Autodesk Fusion 360 part; units mm, degrees
(part 3 of 5)
  line L715 (-40.8866, -85.4677) -> (-40.8866, -98.4677)
  line L716 (118.3697, -66.4177) -> (118.3697, -79.4177)
  arc A698 (151.2072, -3.7177) -> (151.7072, -3.2177) centre (151.2072, -3.2177) ccw
  arc A699 (22.6197, -79.9177) -> (23.1197, -79.4177) centre (22.6197, -79.4177) ccw
  arc A700 (-80.4246, -67.4177) -> (-80.9246, -66.9177) centre (-80.9246, -67.4177) ccw
  line L717 (18.3572, -9.2677) -> (18.3572, -22.2677)
  line L718 (-26.8866, -85.4677) -> (-26.8866, -98.4677)
  arc A701 (155.4629, -62.3677) -> (155.9629, -62.8677) centre (155.9629, -62.3677) ccw
  arc A702 (119.1572, -8.7677) -> (118.6572, -9.2677) centre (119.1572, -9.2677) ccw
  arc A703 (-39.2928, -3.7177) -> (-38.7928, -3.2177) centre (-39.2928, -3.2177) ccw
  line L719 (31.0509, -98.9677) -> (44.0509, -98.9677)
  line L720 (-64.9866, -66.4177) -> (-64.9866, -79.4177)
  line L721 (-87.4246, -67.4177) -> (-87.4246, -81.4177)
  arc A704 (17.8572, -22.7677) -> (18.3572, -22.2677) centre (17.8572, -22.2677) ccw
  arc A705 (-83.7491, -60.3677) -> (-83.2491, -60.8677) centre (-83.2491, -60.3677) ccw
  arc A706 (108.3447, -60.8677) -> (108.8447, -60.3677) centre (108.3447, -60.3677) ccw
  line L722 (176.3072, -65.9177) -> (189.3072, -65.9177)
  line L723 (151.7072, 9.7823) -> (151.7072, -3.2177)
  line L724 (-15.9491, -86.4677) -> (-15.9491, -100.4677)
  arc A707 (-52.2928, -8.7677) -> (-52.7928, -9.2677) centre (-52.2928, -9.2677) ccw
  line L725 (-15.4491, -100.9677) -> (-9.4491, -100.9677)
  line L726 (44.5509, -85.4677) -> (44.5509, -98.4677)
  arc A708 (57.2447, -46.8677) -> (56.7447, -47.3677) centre (57.2447, -47.3677) ccw
  arc A709 (85.3197, -79.4177) -> (85.8197, -79.9177) centre (85.8197, -79.4177) ccw
  line L727 (-48.0303, -66.4177) -> (-48.0303, -79.4177)
  line L728 (80.5572, -9.2677) -> (80.5572, -22.2677)
  arc A710 (-15.4803, -79.9177) -> (-14.9803, -79.4177) centre (-15.4803, -79.4177) ccw
  line L729 (56.4572, -9.2677) -> (56.4572, -22.2677)
  line L730 (138.2072, 10.2823) -> (151.2072, 10.2823)
  arc A711 (-74.5116, -85.4677) -> (-75.0116, -84.9677) centre (-75.0116, -85.4677) ccw
  line L731 (156.7572, 9.7823) -> (156.7572, -3.2177)
  line L732 (47.2197, -66.4177) -> (47.2197, -79.4177)
  arc A712 (9.1197, -79.4177) -> (9.6197, -79.9177) centre (9.6197, -79.4177) ccw
  arc A713 (44.0509, -98.9677) -> (44.5509, -98.4677) centre (44.0509, -98.4677) ccw
  line L733 (-50.6991, -85.4677) -> (-50.6991, -98.4677)
  arc A714 (118.6572, -3.2177) -> (119.1572, -3.7177) centre (119.1572, -3.2177) ccw
  line L734 (100.1072, -8.7677) -> (113.1072, -8.7677)
  line L735 (104.3697, -66.4177) -> (104.3697, -79.4177)
  arc A715 (4.8572, -8.7677) -> (4.3572, -9.2677) centre (4.8572, -9.2677) ccw
  line L736 (186.3389, -48.3677) -> (186.3389, -62.3677)
  arc A716 (99.6072, -3.2177) -> (100.1072, -3.7177) centre (100.1072, -3.2177) ccw
  arc A717 (118.3697, -66.4177) -> (117.8697, -65.9177) centre (117.8697, -66.4177) ccw
  line L737 (28.6697, -65.9177) -> (41.6697, -65.9177)
  arc A718 (60.7197, -79.9177) -> (61.2197, -79.4177) centre (60.7197, -79.4177) ccw
  arc A719 (151.7072, 9.7823) -> (151.2072, 10.2823) centre (151.2072, 9.7823) ccw
  arc A720 (51.1947, -60.8677) -> (51.6947, -60.3677) centre (51.1947, -60.3677) ccw
  arc A721 (117.8697, -79.9177) -> (118.3697, -79.4177) centre (117.8697, -79.4177) ccw
  arc A722 (-40.8866, -98.4677) -> (-40.3866, -98.9677) centre (-40.3866, -98.4677) ccw
  arc A723 (-33.2428, 10.2823) -> (-33.7428, 9.7823) centre (-33.2428, 9.7823) ccw
  arc A724 (66.2697, -79.4177) -> (66.7697, -79.9177) centre (66.7697, -79.4177) ccw
  line L738 (157.2572, 10.2823) -> (170.2572, 10.2823)
  arc A725 (176.3072, -84.9677) -> (175.8072, -85.4677) centre (176.3072, -85.4677) ccw
  arc A726 (-64.1991, -84.9677) -> (-64.6991, -85.4677) centre (-64.1991, -85.4677) ccw
  arc A727 (-64.9866, -66.4177) -> (-65.4866, -65.9177) centre (-65.4866, -66.4177) ccw
  line L739 (-80.4246, -67.4177) -> (-80.4246, -81.4177)
  arc A728 (3.5697, -79.9177) -> (4.0697, -79.4177) centre (3.5697, -79.4177) ccw
  arc A729 (-58.3428, -3.7177) -> (-57.8428, -3.2177) centre (-58.3428, -3.2177) ccw
  arc A730 (-28.4803, -65.9177) -> (-28.9803, -66.4177) centre (-28.4803, -66.4177) ccw
  line L740 (100.1072, -3.7177) -> (113.1072, -3.7177)
  arc A731 (-5.9553, -60.8677) -> (-5.4553, -60.3677) centre (-5.9553, -60.3677) ccw
  arc A732 (-88.0116, -84.9677) -> (-88.5116, -85.4677) centre (-88.0116, -85.4677) ccw
  line L741 (37.4072, -9.2677) -> (37.4072, -22.2677)
  arc A733 (51.6947, -47.3677) -> (51.1947, -46.8677) centre (51.1947, -47.3677) ccw
  arc A734 (19.1447, -46.8677) -> (18.6447, -47.3677) centre (19.1447, -47.3677) ccw
  arc A735 (51.9822, -41.3177) -> (52.4822, -41.8177) centre (52.4822, -41.3177) ccw
  line L742 (99.3197, -66.4177) -> (99.3197, -79.4177)
  line L743 (-19.7428, -9.2677) -> (-19.7428, -22.2677)
  line L744 (47.7197, -65.9177) -> (60.7197, -65.9177)
  line L745 (52.4822, -41.8177) -> (65.4822, -41.8177)
  line L746 (52.4822, -27.8177) -> (65.4822, -27.8177)
  arc A736 (170.2572, -3.7177) -> (170.7572, -3.2177) centre (170.2572, -3.2177) ccw
  line L747 (189.8072, 9.7823) -> (189.8072, -3.2177)
  arc A737 (180.2822, -9.2677) -> (179.7822, -8.7677) centre (179.7822, -9.2677) ccw
  line L748 (208.8572, 9.7823) -> (208.8572, -3.2177)
  arc A738 (208.8572, 9.7823) -> (208.3572, 10.2823) centre (208.3572, 9.7823) ccw
  arc A739 (195.3572, 10.2823) -> (194.8572, 9.7823) centre (195.3572, 9.7823) ccw
  arc A740 (182.2202, -9.7677) -> (181.7202, -10.2677) centre (182.2202, -10.2677) ccw
  arc A741 (208.3572, -3.7177) -> (208.8572, -3.2177) centre (208.3572, -3.2177) ccw
  line L749 (195.3572, 10.2823) -> (208.3572, 10.2823)
  line L750 (195.3572, -3.7177) -> (208.3572, -3.7177)
  line L751 (176.3072, -3.7177) -> (189.3072, -3.7177)
  line L752 (176.3072, 10.2823) -> (189.3072, 10.2823)
  arc A742 (175.8072, -3.2177) -> (176.3072, -3.7177) centre (176.3072, -3.2177) ccw
  arc A743 (195.3572, -8.7677) -> (194.8572, -9.2677) centre (195.3572, -9.2677) ccw
  arc A744 (176.3072, 10.2823) -> (175.8072, 9.7823) centre (176.3072, 9.7823) ccw
  line L753 (195.3572, -8.7677) -> (208.3572, -8.7677)
  arc A745 (170.7572, 9.7823) -> (170.2572, 10.2823) centre (170.2572, 9.7823) ccw
  arc A746 (177.9009, -47.3677) -> (177.4009, -46.8677) centre (177.4009, -47.3677) ccw
  arc A747 (208.8572, -28.3177) -> (208.3572, -27.8177) centre (208.3572, -28.3177) ccw
  arc A748 (171.5447, -27.8177) -> (171.0447, -28.3177) centre (171.5447, -28.3177) ccw
  line L754 (146.9447, -47.3677) -> (146.9447, -60.3677)
  arc A749 (188.2202, -24.7677) -> (188.7202, -24.2677) centre (188.2202, -24.2677) ccw
  line L755 (171.0447, -28.3177) -> (171.0447, -41.3177)
  line L756 (-5.4553, -47.3677) -> (-5.4553, -60.3677)
  arc A750 (195.3572, -27.8177) -> (194.8572, -28.3177) centre (195.3572, -28.3177) ccw
  arc A751 (162.4629, -48.3677) -> (161.9629, -47.8677) centre (161.9629, -48.3677) ccw
  line L757 (208.8572, -9.2677) -> (208.8572, -22.2677)
  line L758 (132.9447, -47.3677) -> (132.9447, -60.3677)
  arc A752 (195.3572, -46.8677) -> (194.8572, -47.3677) centre (195.3572, -47.3677) ccw
  line L759 (180.2822, -9.2677) -> (180.2822, -22.2677)
  arc A753 (186.3389, -48.3677) -> (185.8389, -47.8677) centre (185.8389, -48.3677) ccw
  line L760 (181.7202, -10.2677) -> (181.7202, -24.2677)
  line L761 (-24.5053, -47.3677) -> (-24.5053, -60.3677)
  line L762 (-113.7226, -118.8427) -> (-113.7226, 57.4273)
  line L763 (42.9572, 10.2823) -> (55.9572, 10.2823)
  line L764 (188.7202, -10.2677) -> (188.7202, -24.2677)
  arc A754 (37.4072, -9.2677) -> (36.9072, -8.7677) centre (36.9072, -9.2677) ccw
  line L765 (-43.5553, -47.3677) -> (-43.5553, -60.3677)
  line L766 (194.8572, -9.2677) -> (194.8572, -22.2677)
  line L767 (75.7947, -47.3677) -> (75.7947, -60.3677)
  line L768 (-57.5553, -47.3677) -> (-57.5553, -60.3677)
  line L769 (194.8572, -47.3677) -> (194.8572, -60.3677)
  line L770 (42.9572, -3.7177) -> (55.9572, -3.7177)
  line L771 (177.9009, -47.3677) -> (177.9009, -60.3677)
  arc A755 (55.9572, -3.7177) -> (56.4572, -3.2177) centre (55.9572, -3.2177) ccw
  arc A756 (56.4572, 9.7823) -> (55.9572, 10.2823) centre (55.9572, 9.7823) ccw
  arc A757 (17.8572, -3.7177) -> (18.3572, -3.2177) centre (17.8572, -3.2177) ccw
  line L772 (194.8572, 9.7823) -> (194.8572, -3.2177)
  arc A758 (194.8572, -3.2177) -> (195.3572, -3.7177) centre (195.3572, -3.2177) ccw
  line L773 (175.8072, 9.7823) -> (175.8072, -3.2177)
  arc A759 (188.7202, -10.2677) -> (188.2202, -9.7677) centre (188.2202, -10.2677) ccw
  arc A760 (208.8572, -47.3677) -> (208.3572, -46.8677) centre (208.3572, -47.3677) ccw
  line L774 (171.5447, -27.8177) -> (184.5447, -27.8177)
  arc A761 (179.7822, -22.7677) -> (180.2822, -22.2677) centre (179.7822, -22.2677) ccw
  line L775 (163.9009, -47.3677) -> (163.9009, -60.3677)
  line L776 (195.3572, -46.8677) -> (208.3572, -46.8677)
  line L777 (94.8447, -47.3677) -> (94.8447, -60.3677)
  line L778 (182.2202, -24.7677) -> (188.2202, -24.7677)
  line L779 (179.8389, -47.8677) -> (185.8389, -47.8677)
  line L780 (208.8572, -28.3177) -> (208.8572, -41.3177)
  arc A762 (184.5447, -41.8177) -> (185.0447, -41.3177) centre (184.5447, -41.3177) ccw
  arc A763 (185.0447, -28.3177) -> (184.5447, -27.8177) centre (184.5447, -28.3177) ccw
  arc A764 (189.3072, -3.7177) -> (189.8072, -3.2177) centre (189.3072, -3.2177) ccw
  arc A765 (189.8072, 9.7823) -> (189.3072, 10.2823) centre (189.3072, 9.7823) ccw
  line L781 (182.2202, -9.7677) -> (188.2202, -9.7677)
  line L782 (47.7197, -79.9177) -> (60.7197, -79.9177)
  line L783 (57.2447, -46.8677) -> (70.2447, -46.8677)
  line L784 (-113.7226, 57.4273) -> (228.9474, 57.4273)
  line L785 (18.6447, -47.3677) -> (18.6447, -60.3677)
  line L786 (89.7947, -47.3677) -> (89.7947, -60.3677)
  arc A766 (36.9072, -3.7177) -> (37.4072, -3.2177) centre (36.9072, -3.2177) ccw
  arc A767 (42.9572, -8.7677) -> (42.4572, -9.2677) centre (42.9572, -9.2677) ccw
  line L787 (56.7447, -47.3677) -> (56.7447, -60.3677)
  line L788 (51.6947, -47.3677) -> (51.6947, -60.3677)
  line L789 (-0.4053, -47.3677) -> (-0.4053, -60.3677)
  line L790 (208.8572, -47.3677) -> (208.8572, -60.3677)
  arc A768 (37.4072, 9.7823) -> (36.9072, 10.2823) centre (36.9072, 9.7823) ccw
  line L791 (13.5947, -47.3677) -> (13.5947, -60.3677)
  line L792 (-83.7491, -47.3677) -> (-83.7491, -60.3677)
  line L793 (-38.5053, -47.3677) -> (-38.5053, -60.3677)
  line L794 (127.8947, -47.3677) -> (127.8947, -60.3677)
  line L795 (37.6947, -47.3677) -> (37.6947, -60.3677)
  arc A769 (23.9072, -8.7677) -> (23.4072, -9.2677) centre (23.9072, -9.2677) ccw
  arc A770 (179.8389, -47.8677) -> (179.3389, -48.3677) centre (179.8389, -48.3677) ccw
  line L796 (70.7447, -47.3677) -> (70.7447, -60.3677)
  line L797 (-19.4553, -47.3677) -> (-19.4553, -60.3677)
  arc A771 (56.4572, -9.2677) -> (55.9572, -8.7677) centre (55.9572, -9.2677) ccw
  line L798 (113.8947, -47.3677) -> (113.8947, -60.3677)
  arc A772 (23.9072, 10.2823) -> (23.4072, 9.7823) centre (23.9072, 9.7823) ccw
  line L799 (108.8447, -47.3677) -> (108.8447, -60.3677)
  line L800 (-69.7491, -47.3677) -> (-69.7491, -60.3677)
  line L801 (32.6447, -47.3677) -> (32.6447, -60.3677)
  line L802 (-18.9553, -60.8677) -> (-5.9553, -60.8677)
  line L803 (-23.7178, -27.8177) -> (-10.7178, -27.8177)
  line L804 (228.9474, 57.4273) -> (228.9474, -118.8427)
  arc A773 (18.3572, -9.2677) -> (17.8572, -8.7677) centre (17.8572, -9.2677) ccw
  line L805 (-28.4803, -65.9177) -> (-15.4803, -65.9177)
  line L806 (-33.2428, 10.2823) -> (-20.2428, 10.2823)
  arc A774 (42.4572, -3.2177) -> (42.9572, -3.7177) centre (42.9572, -3.2177) ccw
  line L807 (23.9072, -8.7677) -> (36.9072, -8.7677)
  line L808 (-33.2428, -8.7677) -> (-20.2428, -8.7677)
  line L809 (42.4572, 9.7823) -> (42.4572, -3.2177)
  line L810 (-23.7178, -41.8177) -> (-10.7178, -41.8177)
  line L811 (18.3572, 9.7823) -> (18.3572, -3.2177)
  line L812 (119.1572, -8.7677) -> (132.1572, -8.7677)
  arc A775 (155.9629, -47.8677) -> (155.4629, -48.3677) centre (155.9629, -48.3677) ccw
  line L813 (-28.4803, -79.9177) -> (-15.4803, -79.9177)
  line L814 (123.9197, -79.9177) -> (136.9197, -79.9177)
  line L815 (-57.0553, -60.8677) -> (-44.0553, -60.8677)
  line L816 (128.6822, -27.8177) -> (141.6822, -27.8177)
  line L817 (-64.1991, -98.9677) -> (-51.1991, -98.9677)
  line L818 (-64.1991, -84.9677) -> (-51.1991, -84.9677)
  line L819 (128.6822, -41.8177) -> (141.6822, -41.8177)
  line L820 (42.9572, -8.7677) -> (55.9572, -8.7677)
  line L821 (9.6197, -79.9177) -> (22.6197, -79.9177)
  line L822 (19.1447, -60.8677) -> (32.1447, -60.8677)
  line L823 (-33.2428, -22.7677) -> (-20.2428, -22.7677)
  line L824 (133.4447, -60.8677) -> (146.4447, -60.8677)
  arc A776 (157.2572, 10.2823) -> (156.7572, 9.7823) centre (157.2572, 9.7823) ccw
  line L825 (123.9197, -65.9177) -> (136.9197, -65.9177)
  line L826 (9.6197, -65.9177) -> (22.6197, -65.9177)
  line L827 (119.1572, -22.7677) -> (132.1572, -22.7677)
  line L828 (119.1572, -3.7177) -> (132.1572, -3.7177)
  line L829 (28.6697, -79.9177) -> (41.6697, -79.9177)
  line L830 (119.1572, 10.2823) -> (132.1572, 10.2823)
  line L831 (85.8197, -65.9177) -> (98.8197, -65.9177)
  line L832 (37.4072, 9.7823) -> (37.4072, -3.2177)
  line L833 (138.2072, -8.7677) -> (151.2072, -8.7677)
  line L834 (4.8572, -8.7677) -> (17.8572, -8.7677)
  line L835 (-9.4303, -79.9177) -> (3.5697, -79.9177)
  line L836 (-9.9303, -66.4177) -> (-9.9303, -79.4177)
  arc A777 (-44.0553, -60.8677) -> (-43.5553, -60.3677) centre (-44.0553, -60.3677) ccw
  line L837 (-78.9866, -66.4177) -> (-78.9866, -79.4177)
  line L838 (-15.4491, -85.9677) -> (-9.4491, -85.9677)
  line L839 (-86.9246, -66.9177) -> (-80.9246, -66.9177)
  arc A778 (132.6572, -9.2677) -> (132.1572, -8.7677) centre (132.1572, -9.2677) ccw
  arc A779 (85.8197, -65.9177) -> (85.3197, -66.4177) centre (85.8197, -66.4177) ccw
  arc A780 (-64.6991, -98.4677) -> (-64.1991, -98.9677) centre (-64.1991, -98.4677) ccw
  arc A781 (28.1697, -79.4177) -> (28.6697, -79.9177) centre (28.6697, -79.4177) ccw
  arc A782 (-56.5486, -67.4177) -> (-57.0486, -66.9177) centre (-57.0486, -67.4177) ccw
  arc A783 (56.7447, -60.3677) -> (57.2447, -60.8677) centre (57.2447, -60.3677) ccw
  line L840 (-71.3428, 10.2823) -> (-58.3428, 10.2823)
  line L841 (-9.4303, -65.9177) -> (3.5697, -65.9177)
  arc A784 (156.7572, -3.2177) -> (157.2572, -3.7177) centre (157.2572, -3.2177) ccw
  line L842 (4.8572, 10.2823) -> (17.8572, 10.2823)
  line L843 (31.0509, -84.9677) -> (44.0509, -84.9677)
  line L844 (-88.0116, -98.9677) -> (-75.0116, -98.9677)
  arc A785 (32.1447, -60.8677) -> (32.6447, -60.3677) centre (32.1447, -60.3677) ccw
  arc A786 (44.5509, -85.4677) -> (44.0509, -84.9677) centre (44.0509, -85.4677) ccw
  line L845 (56.4572, 9.7823) -> (56.4572, -3.2177)
  arc A787 (189.3072, -79.9177) -> (189.8072, -79.4177) centre (189.3072, -79.4177) ccw
  arc A788 (-28.9803, -79.4177) -> (-28.4803, -79.9177) centre (-28.4803, -79.4177) ccw
  line L846 (28.1697, -66.4177) -> (28.1697, -79.4177)
  arc A789 (175.8072, -79.4177) -> (176.3072, -79.9177) centre (176.3072, -79.4177) ccw
  arc A790 (66.7697, -65.9177) -> (66.2697, -66.4177) centre (66.7697, -66.4177) ccw
  arc A791 (99.3197, -66.4177) -> (98.8197, -65.9177) centre (98.8197, -66.4177) ccw
  arc A792 (47.2197, -79.4177) -> (47.7197, -79.9177) centre (47.7197, -79.4177) ccw
  line L847 (23.4072, -9.2677) -> (23.4072, -22.2677)
  line L848 (-47.5303, -65.9177) -> (-34.5303, -65.9177)
  arc A793 (37.6947, -60.3677) -> (38.1947, -60.8677) centre (38.1947, -60.3677) ccw
  arc A794 (23.1197, -66.4177) -> (22.6197, -65.9177) centre (22.6197, -66.4177) ccw
  arc A795 (137.7072, -3.2177) -> (138.2072, -3.7177) centre (138.2072, -3.2177) ccw
  arc A796 (208.3572, -79.9177) -> (208.8572, -79.4177) centre (208.3572, -79.4177) ccw
  arc A797 (-63.0486, -66.9177) -> (-63.5486, -67.4177) centre (-63.0486, -67.4177) ccw
  line L849 (99.6072, -9.2677) -> (99.6072, -22.2677)
  line L850 (30.5509, -85.4677) -> (30.5509, -98.4677)
  arc A798 (194.8572, -79.4177) -> (195.3572, -79.9177) centre (195.3572, -79.4177) ccw
  arc A799 (31.0509, -84.9677) -> (30.5509, -85.4677) centre (31.0509, -85.4677) ccw
  arc A800 (-86.9246, -66.9177) -> (-87.4246, -67.4177) centre (-86.9246, -67.4177) ccw
  arc A801 (-14.9803, -66.4177) -> (-15.4803, -65.9177) centre (-15.4803, -66.4177) ccw
  line L851 (-28.9803, -66.4177) -> (-28.9803, -79.4177)
  line L852 (138.2072, -3.7177) -> (151.2072, -3.7177)
  line L853 (0.0947, -60.8677) -> (13.0947, -60.8677)
  arc A802 (-75.0116, -98.9677) -> (-74.5116, -98.4677) centre (-75.0116, -98.4677) ccw
  arc A803 (42.1697, -66.4177) -> (41.6697, -65.9177) centre (41.6697, -66.4177) ccw
  arc A804 (158.3442, -9.7677) -> (157.8442, -10.2677) centre (158.3442, -10.2677) ccw
  arc A805 (132.9447, -60.3677) -> (133.4447, -60.8677) centre (133.4447, -60.3677) ccw
  line L854 (-63.0486, -81.9177) -> (-57.0486, -81.9177)
  line L855 (-14.6928, -9.2677) -> (-14.6928, -22.2677)
  line L856 (-88.5116, -85.4677) -> (-88.5116, -98.4677)
  line L857 (164.4009, -46.8677) -> (177.4009, -46.8677)
  line L858 (-86.9246, -81.9177) -> (-80.9246, -81.9177)
  line L859 (23.1197, -66.4177) -> (23.1197, -79.4177)
  arc A806 (-0.4053, -60.3677) -> (0.0947, -60.8677) centre (0.0947, -60.3677) ccw
  arc A807 (98.8197, -79.9177) -> (99.3197, -79.4177) centre (98.8197, -79.4177) ccw
  line L860 (61.5072, -9.2677) -> (61.5072, -22.2677)
  line L861 (-64.6991, -85.4677) -> (-64.6991, -98.4677)
  arc A808 (-65.4866, -79.9177) -> (-64.9866, -79.4177) centre (-65.4866, -79.4177) ccw
  arc A809 (132.6572, 9.7823) -> (132.1572, 10.2823) centre (132.1572, 9.7823) ccw
  arc A810 (-27.3866, -98.9677) -> (-26.8866, -98.4677) centre (-27.3866, -98.4677) ccw
  arc A811 (47.7197, -65.9177) -> (47.2197, -66.4177) centre (47.7197, -66.4177) ccw
  arc A812 (138.2072, -8.7677) -> (137.7072, -9.2677) centre (138.2072, -9.2677) ccw
  arc A813 (18.3572, 9.7823) -> (17.8572, 10.2823) centre (17.8572, 9.7823) ccw
  arc A814 (28.6697, -65.9177) -> (28.1697, -66.4177) centre (28.6697, -66.4177) ccw
  line L862 (-71.3428, -8.7677) -> (-58.3428, -8.7677)
  line L863 (-71.3428, -3.7177) -> (-58.3428, -3.7177)
  arc A815 (42.9572, 10.2823) -> (42.4572, 9.7823) centre (42.9572, 9.7823) ccw
  line L864 (164.4009, -60.8677) -> (177.4009, -60.8677)
  line L865 (81.0572, 10.2823) -> (94.0572, 10.2823)
  line L866 (157.2572, -3.7177) -> (170.2572, -3.7177)
  line L867 (81.0572, -8.7677) -> (94.0572, -8.7677)
  line L868 (38.1947, -60.8677) -> (51.1947, -60.8677)
  arc A816 (132.1572, -3.7177) -> (132.6572, -3.2177) centre (132.1572, -3.2177) ccw
  arc A817 (-87.4246, -81.4177) -> (-86.9246, -81.9177) centre (-86.9246, -81.4177) ccw
  arc A818 (164.8442, -10.2677) -> (164.3442, -9.7677) centre (164.3442, -10.2677) ccw
  arc A819 (-8.9491, -86.4677) -> (-9.4491, -85.9677) centre (-9.4491, -86.4677) ccw
  arc A820 (13.0947, -60.8677) -> (13.5947, -60.3677) centre (13.0947, -60.3677) ccw
  line L869 (95.3447, -60.8677) -> (108.3447, -60.8677)
  line L870 (-38.0053, -60.8677) -> (-25.0053, -60.8677)
  arc A821 (-80.9246, -81.9177) -> (-80.4246, -81.4177) centre (-80.9246, -81.4177) ccw
  line L871 (90.5822, -27.8177) -> (103.5822, -27.8177)
  arc A822 (-57.0486, -81.9177) -> (-56.5486, -81.4177) centre (-57.0486, -81.4177) ccw
  line L872 (166.7822, -8.7677) -> (179.7822, -8.7677)
  line L873 (-33.2428, -3.7177) -> (-20.2428, -3.7177)
  line L874 (132.6572, 9.7823) -> (132.6572, -3.2177)
  line L875 (23.4072, 9.7823) -> (23.4072, -3.2177)
  line L876 (-61.8178, -27.8177) -> (-48.8178, -27.8177)
  line L877 (81.0572, -3.7177) -> (94.0572, -3.7177)
  line L878 (23.9072, -3.7177) -> (36.9072, -3.7177)
  arc A823 (41.6697, -79.9177) -> (42.1697, -79.4177) centre (41.6697, -79.4177) ccw
  line L879 (90.5822, -41.8177) -> (103.5822, -41.8177)
  arc A824 (-63.5486, -81.4177) -> (-63.0486, -81.9177) centre (-63.0486, -81.4177) ccw
  line L880 (-40.3866, -98.9677) -> (-27.3866, -98.9677)
  arc A825 (-25.0053, -60.8677) -> (-24.5053, -60.3677) centre (-25.0053, -60.3677) ccw
  line L881 (137.7072, 9.7823) -> (137.7072, -3.2177)
  line L882 (4.8572, -3.7177) -> (17.8572, -3.7177)
  line L883 (14.3822, -41.8177) -> (27.3822, -41.8177)
  line L884 (4.8572, -22.7677) -> (17.8572, -22.7677)
  arc A826 (23.4072, -3.2177) -> (23.9072, -3.7177) centre (23.9072, -3.2177) ccw
  line L885 (-47.5303, -79.9177) -> (-34.5303, -79.9177)
  line L886 (85.8197, -79.9177) -> (98.8197, -79.9177)
  line L887 (81.0572, -22.7677) -> (94.0572, -22.7677)
  line L888 (-56.5486, -67.4177) -> (-56.5486, -81.4177)
  arc A827 (-9.9303, -79.4177) -> (-9.4303, -79.9177) centre (-9.4303, -79.4177) ccw
  line L889 (23.9072, 10.2823) -> (36.9072, 10.2823)
  line L890 (-34.0303, -66.4177) -> (-34.0303, -79.4177)
  line L891 (14.3822, -27.8177) -> (27.3822, -27.8177)
  arc A828 (194.8572, -41.3177) -> (195.3572, -41.8177) centre (195.3572, -41.3177) ccw
  arc A829 (194.8572, -22.2677) -> (195.3572, -22.7677) centre (195.3572, -22.2677) ccw
  line L892 (194.8572, -28.3177) -> (194.8572, -41.3177)
  line L893 (195.3572, -22.7677) -> (208.3572, -22.7677)
  arc A830 (208.3572, -41.8177) -> (208.8572, -41.3177) centre (208.3572, -41.3177) ccw
  line L894 (185.0447, -28.3177) -> (185.0447, -41.3177)
  line L895 (195.3572, -41.8177) -> (208.3572, -41.8177)
  arc A831 (181.7202, -24.2677) -> (182.2202, -24.7677) centre (182.2202, -24.2677) ccw
  arc A832 (208.3572, -22.7677) -> (208.8572, -22.2677) centre (208.3572, -22.2677) ccw
  line L896 (171.5447, -41.8177) -> (184.5447, -41.8177)
  arc A833 (171.0447, -41.3177) -> (171.5447, -41.8177) centre (171.5447, -41.3177) ccw
  line L897 (195.3572, -27.8177) -> (208.3572, -27.8177)
  line L898 (57.2447, -60.8677) -> (70.2447, -60.8677)
  line L899 (228.9474, -118.8427) -> (-113.7226, -118.8427)
  line L900 (123.1322, -28.3177) -> (123.1322, -41.3177)
  arc A834 (114.3947, -46.8677) -> (113.8947, -47.3677) centre (114.3947, -47.3677) ccw
  line L901 (156.7572, -85.4677) -> (156.7572, -98.4677)
  line L902 (151.7072, -85.4677) -> (151.7072, -98.4677)
  arc A835 (-71.8428, -22.2677) -> (-71.3428, -22.7677) centre (-71.3428, -22.2677) ccw
  line L903 (-57.0553, -46.8677) -> (-44.0553, -46.8677)
  arc A836 (-69.7491, -47.3677) -> (-70.2491, -46.8677) centre (-70.2491, -47.3677) ccw
  arc A837 (-90.8928, -22.2677) -> (-90.3928, -22.7677) centre (-90.3928, -22.2677) ccw
  arc A838 (170.2572, -98.9677) -> (170.7572, -98.4677) centre (170.2572, -98.4677) ccw
  arc A839 (-86.1303, -41.3177) -> (-85.6303, -41.8177) centre (-85.6303, -41.3177) ccw
  arc A840 (149.6134, -79.4177) -> (150.1134, -79.9177) centre (150.1134, -79.4177) ccw
  arc A841 (-85.6303, -27.8177) -> (-86.1303, -28.3177) centre (-85.6303, -28.3177) ccw
  line L904 (8.8322, -28.3177) -> (8.8322, -41.3177)
  arc A842 (-77.3928, -22.7677) -> (-76.8928, -22.2677) centre (-77.3928, -22.2677) ccw
  line L905 (95.3447, -46.8677) -> (108.3447, -46.8677)
  line L906 (-29.2678, -28.3177) -> (-29.2678, -41.3177)
  arc A843 (-38.0053, -46.8677) -> (-38.5053, -47.3677) centre (-38.0053, -47.3677) ccw
  line L907 (-85.6303, -27.8177) -> (-72.6303, -27.8177)
  arc A844 (163.1134, -79.9177) -> (163.6134, -79.4177) centre (163.1134, -79.4177) ccw
  arc A845 (-33.7428, -22.2677) -> (-33.2428, -22.7677) centre (-33.2428, -22.2677) ccw
  line L908 (114.3947, -46.8677) -> (127.3947, -46.8677)
  arc A846 (14.3822, -27.8177) -> (13.8822, -28.3177) centre (14.3822, -28.3177) ccw
  arc A847 (-58.3428, -22.7677) -> (-57.8428, -22.2677) centre (-58.3428, -22.2677) ccw
  arc A848 (161.9629, -62.8677) -> (162.4629, -62.3677) centre (161.9629, -62.3677) ccw
  line L909 (-85.6303, -41.8177) -> (-72.6303, -41.8177)
  arc A849 (-42.7678, -27.8177) -> (-43.2678, -28.3177) centre (-42.7678, -28.3177) ccw
  arc A850 (163.9009, -60.3677) -> (164.4009, -60.8677) centre (164.4009, -60.3677) ccw
  line L910 (-18.9553, -46.8677) -> (-5.9553, -46.8677)
  arc A851 (-29.2678, -28.3177) -> (-29.7678, -27.8177) centre (-29.7678, -28.3177) ccw
  arc A852 (-4.6678, -27.8177) -> (-5.1678, -28.3177) centre (-4.6678, -28.3177) ccw
  line L911 (137.4197, -66.4177) -> (137.4197, -79.4177)
  line L912 (163.6134, -66.4177) -> (163.6134, -79.4177)
  arc A853 (-83.2491, -46.8677) -> (-83.7491, -47.3677) centre (-83.2491, -47.3677) ccw
  arc A854 (146.4447, -60.8677) -> (146.9447, -60.3677) centre (146.4447, -60.3677) ccw
  line L913 (170.7572, -85.4677) -> (170.7572, -98.4677)
  line L914 (157.2572, -84.9677) -> (170.2572, -84.9677)
  arc A855 (-39.2928, -22.7677) -> (-38.7928, -22.2677) centre (-39.2928, -22.2677) ccw
  arc A856 (-24.2178, -41.3177) -> (-23.7178, -41.8177) centre (-23.7178, -41.3177) ccw
  arc A857 (-29.7678, -41.8177) -> (-29.2678, -41.3177) centre (-29.7678, -41.3177) ccw
  arc A858 (-48.8178, -41.8177) -> (-48.3178, -41.3177) centre (-48.8178, -41.3177) ccw
  arc A859 (151.2072, -98.9677) -> (151.7072, -98.4677) centre (151.2072, -98.4677) ccw
  arc A860 (-43.5553, -47.3677) -> (-44.0553, -46.8677) centre (-44.0553, -47.3677) ccw
  arc A861 (208.8572, -9.2677) -> (208.3572, -8.7677) centre (208.3572, -9.2677) ccw
  line L915 (170.7572, 9.7823) -> (170.7572, -3.2177)
  arc A862 (-72.1303, -28.3177) -> (-72.6303, -27.8177) centre (-72.6303, -28.3177) ccw
  arc A863 (0.0947, -46.8677) -> (-0.4053, -47.3677) centre (0.0947, -47.3677) ccw
  arc A864 (122.6322, -41.8177) -> (123.1322, -41.3177) centre (122.6322, -41.3177) ccw
  line L916 (13.8822, -28.3177) -> (13.8822, -41.3177)
  line L917 (155.9629, -62.8677) -> (161.9629, -62.8677)
  line L918 (147.7322, -27.8177) -> (160.7322, -27.8177)
  arc A865 (-62.3178, -41.3177) -> (-61.8178, -41.8177) centre (-61.8178, -41.3177) ccw
  line L919 (147.2322, -28.3177) -> (147.2322, -41.3177)
  line L920 (71.5322, -27.8177) -> (84.5322, -27.8177)
  line L921 (133.4447, -46.8677) -> (146.4447, -46.8677)
  line L922 (0.0947, -46.8677) -> (13.0947, -46.8677)
  line L923 (158.3442, -24.7677) -> (164.3442, -24.7677)
  arc A866 (-90.3928, 10.2823) -> (-90.8928, 9.7823) centre (-90.3928, 9.7823) ccw
  line L924 (-90.8928, 9.7823) -> (-90.8928, -3.2177)
  line L925 (-10.2178, -28.3177) -> (-10.2178, -41.3177)
  line L926 (100.1072, -22.7677) -> (113.1072, -22.7677)
  arc A867 (89.7947, -47.3677) -> (89.2947, -46.8677) centre (89.2947, -47.3677) ccw
  line L927 (-90.3928, 10.2823) -> (-77.3928, 10.2823)
  line L928 (-62.3178, -28.3177) -> (-62.3178, -41.3177)
  arc A868 (118.6572, -22.2677) -> (119.1572, -22.7677) centre (119.1572, -22.2677) ccw
  arc A869 (109.1322, -41.3177) -> (109.6322, -41.8177) centre (109.6322, -41.3177) ccw
  arc A870 (123.1322, -28.3177) -> (122.6322, -27.8177) centre (122.6322, -28.3177) ccw
  line L929 (137.7072, -85.4677) -> (137.7072, -98.4677)
  arc A871 (-52.7928, -22.2677) -> (-52.2928, -22.7677) centre (-52.2928, -22.2677) ccw
  line L930 (61.2197, -66.4177) -> (61.2197, -79.4177)
  line L931 (-71.8428, 9.7823) -> (-71.8428, -3.2177)
  line L932 (147.7322, -41.8177) -> (160.7322, -41.8177)
  arc A872 (113.1072, -22.7677) -> (113.6072, -22.2677) centre (113.1072, -22.2677) ccw
  arc A873 (142.1822, -28.3177) -> (141.6822, -27.8177) centre (141.6822, -28.3177) ccw
  line L933 (-43.2678, -28.3177) -> (-43.2678, -41.3177)
  arc A874 (-76.8928, -9.2677) -> (-77.3928, -8.7677) centre (-77.3928, -9.2677) ccw
  arc A875 (-48.3178, -28.3177) -> (-48.8178, -27.8177) centre (-48.8178, -28.3177) ccw
  line L934 (-90.3928, -8.7677) -> (-77.3928, -8.7677)
  arc A876 (104.0822, -28.3177) -> (103.5822, -27.8177) centre (103.5822, -28.3177) ccw
  line L935 (-14.1928, -22.7677) -> (-1.1928, -22.7677)
  arc A877 (156.7572, -98.4677) -> (157.2572, -98.9677) centre (157.2572, -98.4677) ccw
  arc A878 (-43.2678, -41.3177) -> (-42.7678, -41.8177) centre (-42.7678, -41.3177) ccw
  arc A879 (-18.9553, -46.8677) -> (-19.4553, -47.3677) centre (-18.9553, -47.3677) ccw
  arc A880 (-23.7178, -27.8177) -> (-24.2178, -28.3177) centre (-23.7178, -28.3177) ccw
  line L936 (-42.7678, -27.8177) -> (-29.7678, -27.8177)
  line L937 (-90.3928, -3.7177) -> (-77.3928, -3.7177)
  arc A881 (-77.3928, -3.7177) -> (-76.8928, -3.2177) centre (-77.3928, -3.2177) ccw
  arc A882 (13.5947, -47.3677) -> (13.0947, -46.8677) centre (13.0947, -47.3677) ccw
  arc A883 (-90.3928, -8.7677) -> (-90.8928, -9.2677) centre (-90.3928, -9.2677) ccw
  arc A884 (141.6822, -41.8177) -> (142.1822, -41.3177) centre (141.6822, -41.3177) ccw
  arc A885 (-61.8178, -27.8177) -> (-62.3178, -28.3177) centre (-61.8178, -28.3177) ccw
  arc A886 (164.3442, -24.7677) -> (164.8442, -24.2677) centre (164.3442, -24.2677) ccw
  arc A887 (-14.6928, -22.2677) -> (-14.1928, -22.7677) centre (-14.1928, -22.2677) ccw
  arc A888 (94.0572, -22.7677) -> (94.5572, -22.2677) centre (94.0572, -22.2677) ccw
  arc A889 (-90.8928, -3.2177) -> (-90.3928, -3.7177) centre (-90.3928, -3.2177) ccw
  arc A890 (-71.3428, -8.7677) -> (-71.8428, -9.2677) centre (-71.3428, -9.2677) ccw
  line L938 (161.2322, -28.3177) -> (161.2322, -41.3177)
  arc A891 (-72.6303, -41.8177) -> (-72.1303, -41.3177) centre (-72.6303, -41.3177) ccw
  arc A892 (128.6822, -27.8177) -> (128.1822, -28.3177) centre (128.6822, -28.3177) ccw
  arc A893 (170.7572, -85.4677) -> (170.2572, -84.9677) centre (170.2572, -85.4677) ccw
  arc A894 (13.8822, -41.3177) -> (14.3822, -41.8177) centre (14.3822, -41.3177) ccw
  line L939 (109.6322, -27.8177) -> (122.6322, -27.8177)
  line L940 (104.0822, -28.3177) -> (104.0822, -41.3177)
  arc A895 (99.6072, -22.2677) -> (100.1072, -22.7677) centre (100.1072, -22.2677) ccw
  arc A896 (164.4009, -46.8677) -> (163.9009, -47.3677) centre (164.4009, -47.3677) ccw
  line L941 (-90.3928, -22.7677) -> (-77.3928, -22.7677)
  line L942 (-76.8928, 9.7823) -> (-76.8928, -3.2177)
  arc A897 (8.3322, -41.8177) -> (8.8322, -41.3177) centre (8.3322, -41.3177) ccw
  arc A898 (-71.3428, 10.2823) -> (-71.8428, 9.7823) centre (-71.3428, 9.7823) ccw
  line L943 (100.1072, 10.2823) -> (113.1072, 10.2823)
  arc A899 (81.0572, -8.7677) -> (80.5572, -9.2677) centre (81.0572, -9.2677) ccw
  arc A900 (189.3072, -98.9677) -> (189.8072, -98.4677) centre (189.3072, -98.4677) ccw
  line L944 (109.6322, -41.8177) -> (122.6322, -41.8177)
  line L945 (-52.2928, -3.7177) -> (-39.2928, -3.7177)
  line L946 (176.3072, -84.9677) -> (189.3072, -84.9677)
  arc A901 (-19.7428, -9.2677) -> (-20.2428, -8.7677) centre (-20.2428, -9.2677) ccw
  arc A902 (33.4322, -27.8177) -> (32.9322, -28.3177) centre (33.4322, -28.3177) ccw
  line L947 (94.5572, 9.7823) -> (94.5572, -3.2177)
  line L948 (119.1572, -98.9677) -> (132.1572, -98.9677)
  line L949 (-71.3428, -22.7677) -> (-58.3428, -22.7677)
  arc A903 (113.1072, -98.9677) -> (113.6072, -98.4677) centre (113.1072, -98.4677) ccw
  line L950 (42.9572, -22.7677) -> (55.9572, -22.7677)
  arc A904 (62.0072, -8.7677) -> (61.5072, -9.2677) centre (62.0072, -9.2677) ccw
  arc A905 (4.3572, -22.2677) -> (4.8572, -22.7677) centre (4.8572, -22.2677) ccw
  line L951 (132.6572, -9.2677) -> (132.6572, -22.2677)
  line L952 (-38.7928, 9.7823) -> (-38.7928, -3.2177)
  arc A906 (84.0509, -100.4677) -> (84.5509, -100.9677) centre (84.5509, -100.4677) ccw
  line L953 (166.2822, -9.2677) -> (166.2822, -22.2677)
  line L954 (76.2947, -46.8677) -> (89.2947, -46.8677)
  line L955 (194.8572, -66.4177) -> (194.8572, -79.4177)
  arc A907 (85.0322, -28.3177) -> (84.5322, -27.8177) centre (84.5322, -28.3177) ccw
  line L956 (51.9822, -28.3177) -> (51.9822, -41.3177)
  arc A908 (71.0322, -41.3177) -> (71.5322, -41.8177) centre (71.5322, -41.3177) ccw
  arc A909 (89.2947, -60.8677) -> (89.7947, -60.3677) centre (89.2947, -60.3677) ccw
  arc A910 (189.8072, -66.4177) -> (189.3072, -65.9177) centre (189.3072, -66.4177) ccw
  line L957 (23.9072, -22.7677) -> (36.9072, -22.7677)
  arc A911 (-19.7428, 9.7823) -> (-20.2428, 10.2823) centre (-20.2428, 9.7823) ccw
  line L958 (132.6572, -85.4677) -> (132.6572, -98.4677)
  line L959 (189.8072, -85.4677) -> (189.8072, -98.4677)
  line L960 (100.1072, -84.9677) -> (113.1072, -84.9677)
  arc A912 (79.7697, -79.9177) -> (80.2697, -79.4177) centre (79.7697, -79.4177) ccw
  line L961 (-52.2928, 10.2823) -> (-39.2928, 10.2823)
  arc A913 (61.5072, -22.2677) -> (62.0072, -22.7677) centre (62.0072, -22.2677) ccw
  line L962 (162.4629, -48.3677) -> (162.4629, -62.3677)
  line L963 (-14.1928, -3.7177) -> (-1.1928, -3.7177)
  line L964 (155.9629, -47.8677) -> (161.9629, -47.8677)
  line L965 (100.1072, -98.9677) -> (113.1072, -98.9677)
  line L966 (-4.6678, -41.8177) -> (8.3322, -41.8177)
  line L967 (138.2072, -98.9677) -> (151.2072, -98.9677)
  arc A914 (4.3572, -3.2177) -> (4.8572, -3.7177) centre (4.8572, -3.2177) ccw
  arc A915 (75.5072, 9.7823) -> (75.0072, 10.2823) centre (75.0072, 9.7823) ccw
  arc A916 (113.6072, -85.4677) -> (113.1072, -84.9677) centre (113.1072, -85.4677) ccw
  arc A917 (27.8822, -28.3177) -> (27.3822, -27.8177) centre (27.3822, -28.3177) ccw
  line L968 (76.2947, -60.8677) -> (89.2947, -60.8677)
  arc A918 (70.2447, -60.8677) -> (70.7447, -60.3677) centre (70.2447, -60.3677) ccw
  arc A919 (55.9572, -22.7677) -> (56.4572, -22.2677) centre (55.9572, -22.2677) ccw
  line L969 (-57.8428, 9.7823) -> (-57.8428, -3.2177)
  arc A920 (80.2697, -66.4177) -> (79.7697, -65.9177) centre (79.7697, -66.4177) ccw
  arc A921 (-14.6928, -3.2177) -> (-14.1928, -3.7177) centre (-14.1928, -3.2177) ccw
  line L970 (208.8572, -66.4177) -> (208.8572, -79.4177)
  line L971 (-33.7428, 9.7823) -> (-33.7428, -3.2177)
  arc A922 (90.0822, -41.3177) -> (90.5822, -41.8177) centre (90.5822, -41.3177) ccw
  arc A923 (132.1572, -22.7677) -> (132.6572, -22.2677) centre (132.1572, -22.2677) ccw
  arc A924 (95.3447, -46.8677) -> (94.8447, -47.3677) centre (95.3447, -47.3677) ccw
  line L972 (62.0072, -3.7177) -> (75.0072, -3.7177)
  line L973 (66.7697, -65.9177) -> (79.7697, -65.9177)
  line L974 (118.6572, -85.4677) -> (118.6572, -98.4677)
  line L975 (157.8442, -10.2677) -> (157.8442, -24.2677)
  line L976 (-38.7928, -9.2677) -> (-38.7928, -22.2677)
  arc A925 (-1.1928, -3.7177) -> (-0.6928, -3.2177) centre (-1.1928, -3.2177) ccw
  arc A926 (118.6572, -98.4677) -> (119.1572, -98.9677) centre (119.1572, -98.4677) ccw
  line L977 (149.6134, -66.4177) -> (149.6134, -79.4177)
  line L978 (-76.8928, -9.2677) -> (-76.8928, -22.2677)
  arc A927 (161.2322, -28.3177) -> (160.7322, -27.8177) centre (160.7322, -28.3177) ccw
  arc A928 (103.5822, -41.8177) -> (104.0822, -41.3177) centre (103.5822, -41.3177) ccw
  line L979 (61.5072, 9.7823) -> (61.5072, -3.2177)
  arc A929 (80.5572, -3.2177) -> (81.0572, -3.7177) centre (81.0572, -3.2177) ccw
  line L980 (-33.7428, -9.2677) -> (-33.7428, -22.2677)
  arc A930 (195.3572, -65.9177) -> (194.8572, -66.4177) centre (195.3572, -66.4177) ccw
  line L981 (138.2072, -22.7677) -> (151.2072, -22.7677)
  arc A931 (-33.2428, -8.7677) -> (-33.7428, -9.2677) centre (-33.2428, -9.2677) ccw
  line L982 (113.6072, -85.4677) -> (113.6072, -98.4677)
  line L983 (-52.7928, -9.2677) -> (-52.7928, -22.2677)
  arc A932 (70.7447, -47.3677) -> (70.2447, -46.8677) centre (70.2447, -47.3677) ccw
  arc A933 (-38.7928, -9.2677) -> (-39.2928, -8.7677) centre (-39.2928, -9.2677) ccw
  line L984 (80.2697, -66.4177) -> (80.2697, -79.4177)
  line L985 (151.7072, -9.2677) -> (151.7072, -22.2677)
  arc A934 (-10.7178, -41.8177) -> (-10.2178, -41.3177) centre (-10.7178, -41.3177) ccw
  line L986 (-57.8428, -9.2677) -> (-57.8428, -22.2677)
  line L987 (71.0322, -28.3177) -> (71.0322, -41.3177)
  line L988 (195.3572, -65.9177) -> (208.3572, -65.9177)
  line L989 (65.9822, -28.3177) -> (65.9822, -41.3177)
  arc A935 (94.8447, -60.3677) -> (95.3447, -60.8677) centre (95.3447, -60.3677) ccw
  line L990 (62.0072, -8.7677) -> (75.0072, -8.7677)
  line L991 (-19.7428, 9.7823) -> (-19.7428, -3.2177)
  line L992 (-14.1928, -8.7677) -> (-1.1928, -8.7677)
  arc A936 (132.6572, -85.4677) -> (132.1572, -84.9677) centre (132.1572, -85.4677) ccw
  line L993 (-90.8928, -9.2677) -> (-90.8928, -22.2677)
  line L994 (138.2072, -84.9677) -> (151.2072, -84.9677)
  line L995 (62.0072, -22.7677) -> (75.0072, -22.7677)
  arc A937 (4.8572, 10.2823) -> (4.3572, 9.7823) centre (4.8572, 9.7823) ccw
  line L996 (-4.6678, -27.8177) -> (8.3322, -27.8177)
  arc A938 (147.2322, -41.3177) -> (147.7322, -41.8177) centre (147.7322, -41.3177) ccw
  line L997 (150.1134, -79.9177) -> (163.1134, -79.9177)
  arc A939 (128.1822, -41.3177) -> (128.6822, -41.8177) centre (128.6822, -41.3177) ccw
  arc A940 (166.2822, -22.2677) -> (166.7822, -22.7677) centre (166.7822, -22.2677) ccw
  arc A941 (137.4197, -66.4177) -> (136.9197, -65.9177) centre (136.9197, -66.4177) ccw
  arc A942 (-57.0553, -46.8677) -> (-57.5553, -47.3677) centre (-57.0553, -47.3677) ccw
  arc A943 (91.0509, -86.4677) -> (90.5509, -85.9677) centre (90.5509, -86.4677) ccw
  arc A944 (76.2947, -46.8677) -> (75.7947, -47.3677) centre (76.2947, -47.3677) ccw
  arc A945 (108.8447, -47.3677) -> (108.3447, -46.8677) centre (108.3447, -47.3677) ccw
  line L998 (85.0322, -28.3177) -> (85.0322, -41.3177)
  line L999 (84.0509, -86.4677) -> (84.0509, -100.4677)
  arc A946 (137.7072, -22.2677) -> (138.2072, -22.7677) centre (138.2072, -22.2677) ccw
  arc A947 (-5.4553, -47.3677) -> (-5.9553, -46.8677) centre (-5.9553, -47.3677) ccw
  arc A948 (-57.8428, 9.7823) -> (-58.3428, 10.2823) centre (-58.3428, 9.7823) ccw
  line L1000 (66.2697, -66.4177) -> (66.2697, -79.4177)
  arc A949 (-52.7928, -3.2177) -> (-52.2928, -3.7177) centre (-52.2928, -3.2177) ccw
  arc A950 (138.2072, -84.9677) -> (137.7072, -85.4677) centre (138.2072, -85.4677) ccw
  line L1001 (84.5509, -85.9677) -> (90.5509, -85.9677)
  arc A951 (8.8322, -28.3177) -> (8.3322, -27.8177) centre (8.3322, -28.3177) ccw
  line L1002 (164.8442, -10.2677) -> (164.8442, -24.2677)
  line L1003 (-38.0053, -46.8677) -> (-25.0053, -46.8677)
  arc A952 (127.8947, -47.3677) -> (127.3947, -46.8677) centre (127.3947, -47.3677) ccw
  arc A953 (194.8572, -60.3677) -> (195.3572, -60.8677) centre (195.3572, -60.3677) ccw
  line L1004 (104.8697, -79.9177) -> (117.8697, -79.9177)
  line L1005 (119.1572, -84.9677) -> (132.1572, -84.9677)
  arc A954 (-38.7928, 9.7823) -> (-39.2928, 10.2823) centre (-39.2928, 9.7823) ccw
  line L1006 (71.5322, -41.8177) -> (84.5322, -41.8177)
  line L1007 (-71.8428, -9.2677) -> (-71.8428, -22.2677)
  arc A955 (100.1072, -84.9677) -> (99.6072, -85.4677) centre (100.1072, -85.4677) ccw
  line L1008 (-52.2928, -22.7677) -> (-39.2928, -22.7677)
  arc A956 (208.8572, -66.4177) -> (208.3572, -65.9177) centre (208.3572, -66.4177) ccw
  arc A957 (147.7322, -27.8177) -> (147.2322, -28.3177) centre (147.7322, -28.3177) ccw
  arc A958 (61.2197, -66.4177) -> (60.7197, -65.9177) centre (60.7197, -66.4177) ccw
  arc A959 (65.4822, -41.8177) -> (65.9822, -41.3177) centre (65.4822, -41.3177) ccw
  arc A960 (99.6072, -98.4677) -> (100.1072, -98.9677) centre (100.1072, -98.4677) ccw
  arc A961 (119.1572, -84.9677) -> (118.6572, -85.4677) centre (119.1572, -85.4677) ccw
  line L1009 (142.1822, -28.3177) -> (142.1822, -41.3177)
  arc A962 (-5.1678, -41.3177) -> (-4.6678, -41.8177) centre (-4.6678, -41.3177) ccw
  arc A963 (150.1134, -65.9177) -> (149.6134, -66.4177) centre (150.1134, -66.4177) ccw
  arc A964 (151.2072, -22.7677) -> (151.7072, -22.2677) centre (151.2072, -22.2677) ccw
  arc A965 (-71.8428, -3.2177) -> (-71.3428, -3.7177) centre (-71.3428, -3.2177) ccw
  arc A966 (157.8442, -24.2677) -> (158.3442, -24.7677) centre (158.3442, -24.2677) ccw
  arc A967 (146.9447, -47.3677) -> (146.4447, -46.8677) centre (146.4447, -47.3677) ccw
  arc A968 (-1.1928, -22.7677) -> (-0.6928, -22.2677) centre (-1.1928, -22.2677) ccw
  line L1010 (-72.1303, -28.3177) -> (-72.1303, -41.3177)
  line L1011 (128.1822, -28.3177) -> (128.1822, -41.3177)
  arc A969 (-10.2178, -28.3177) -> (-10.7178, -27.8177) centre (-10.7178, -28.3177) ccw
  line L1012 (109.1322, -28.3177) -> (109.1322, -41.3177)
  line L1013 (-83.2491, -46.8677) -> (-70.2491, -46.8677)
  arc A970 (109.6322, -27.8177) -> (109.1322, -28.3177) centre (109.6322, -28.3177) ccw
  arc A971 (160.7322, -41.8177) -> (161.2322, -41.3177) centre (160.7322, -41.3177) ccw
  line L1014 (-86.1303, -28.3177) -> (-86.1303, -41.3177)
  arc A972 (71.5322, -27.8177) -> (71.0322, -28.3177) centre (71.5322, -28.3177) ccw
  arc A973 (90.5509, -100.9677) -> (91.0509, -100.4677) centre (90.5509, -100.4677) ccw
  arc A974 (-20.2428, -22.7677) -> (-19.7428, -22.2677) centre (-20.2428, -22.2677) ccw
  arc A975 (84.5322, -41.8177) -> (85.0322, -41.3177) centre (84.5322, -41.3177) ccw
  line L1015 (-5.1678, -28.3177) -> (-5.1678, -41.3177)
  line L1016 (-42.7678, -41.8177) -> (-29.7678, -41.8177)
  arc A976 (-76.8928, 9.7823) -> (-77.3928, 10.2823) centre (-77.3928, 9.7823) ccw
  line L1017 (155.4629, -48.3677) -> (155.4629, -62.3677)
  arc A977 (-24.5053, -47.3677) -> (-25.0053, -46.8677) centre (-25.0053, -47.3677) ccw
  line L1018 (-48.3178, -28.3177) -> (-48.3178, -41.3177)
  arc A978 (133.4447, -46.8677) -> (132.9447, -47.3677) centre (133.4447, -47.3677) ccw
  line L1019 (-24.2178, -28.3177) -> (-24.2178, -41.3177)
  arc A979 (18.6447, -60.3677) -> (19.1447, -60.8677) centre (19.1447, -60.3677) ccw
  arc A980 (177.4009, -60.8677) -> (177.9009, -60.3677) centre (177.4009, -60.3677) ccw
  line L1020 (75.5072, 9.7823) -> (75.5072, -3.2177)
  arc A981 (-33.7428, -3.2177) -> (-33.2428, -3.7177) centre (-33.2428, -3.2177) ccw
  line L1021 (-0.6928, -9.2677) -> (-0.6928, -22.2677)
  line L1022 (91.0509, -86.4677) -> (91.0509, -100.4677)
  arc A982 (32.9322, -41.3177) -> (33.4322, -41.8177) centre (33.4322, -41.3177) ccw
  line L1023 (195.3572, -84.9677) -> (208.3572, -84.9677)
  line L1024 (195.3572, -79.9177) -> (208.3572, -79.9177)
  arc A983 (151.7072, -9.2677) -> (151.2072, -8.7677) centre (151.2072, -9.2677) ccw
  line L1025 (-78.4866, -79.9177) -> (-65.4866, -79.9177)
  arc A984 (138.2072, 10.2823) -> (137.7072, 9.7823) centre (138.2072, 9.7823) ccw
  arc A985 (175.8072, -98.4677) -> (176.3072, -98.9677) centre (176.3072, -98.4677) ccw
  arc A986 (94.0572, -3.7177) -> (94.5572, -3.2177) centre (94.0572, -3.2177) ccw
  arc A987 (104.8697, -65.9177) -> (104.3697, -66.4177) centre (104.8697, -66.4177) ccw
  arc A988 (-0.6928, -9.2677) -> (-1.1928, -8.7677) centre (-1.1928, -9.2677) ccw
  arc A989 (163.6134, -66.4177) -> (163.1134, -65.9177) centre (163.1134, -66.4177) ccw
  line L1026 (-40.3866, -84.9677) -> (-27.3866, -84.9677)
  line L1027 (9.1197, -66.4177) -> (9.1197, -79.4177)
  line L1028 (118.6572, 9.7823) -> (118.6572, -3.2177)
  line L1029 (179.3389, -48.3677) -> (179.3389, -62.3677)
  line L1030 (32.9322, -28.3177) -> (32.9322, -41.3177)
  line L1031 (208.8572, -85.4677) -> (208.8572, -98.4677)
  line L1032 (-14.9803, -66.4177) -> (-14.9803, -79.4177)
  arc A990 (137.7072, -98.4677) -> (138.2072, -98.9677) centre (138.2072, -98.4677) ccw
  line L1033 (189.8072, -66.4177) -> (189.8072, -79.4177)
  line L1034 (123.4197, -66.4177) -> (123.4197, -79.4177)
  arc A991 (104.3697, -79.4177) -> (104.8697, -79.9177) centre (104.8697, -79.4177) ccw
  arc A992 (36.9072, -22.7677) -> (37.4072, -22.2677) centre (36.9072, -22.2677) ccw
  line L1035 (-52.7928, 9.7823) -> (-52.7928, -3.2177)
  line L1036 (42.4572, -9.2677) -> (42.4572, -22.2677)
  arc A993 (90.5822, -27.8177) -> (90.0822, -28.3177) centre (90.5822, -28.3177) ccw
  arc A994 (208.3572, -98.9677) -> (208.8572, -98.4677) centre (208.3572, -98.4677) ccw
  arc A995 (151.7072, -85.4677) -> (151.2072, -84.9677) centre (151.2072, -85.4677) ccw
  arc A996 (166.7822, -8.7677) -> (166.2822, -9.2677) centre (166.7822, -9.2677) ccw
  arc A997 (-9.4491, -100.9677) -> (-8.9491, -100.4677) centre (-9.4491, -100.4677) ccw
  arc A998 (-26.8866, -85.4677) -> (-27.3866, -84.9677) centre (-27.3866, -85.4677) ccw
  line L1037 (19.1447, -46.8677) -> (32.1447, -46.8677)
  line L1038 (104.8697, -65.9177) -> (117.8697, -65.9177)
  arc A999 (-78.9866, -79.4177) -> (-78.4866, -79.9177) centre (-78.4866, -79.4177) ccw
  line L1039 (33.4322, -41.8177) -> (46.4322, -41.8177)
  arc A1000 (208.3572, -60.8677) -> (208.8572, -60.3677) centre (208.3572, -60.3677) ccw
  line L1040 (-78.4866, -65.9177) -> (-65.4866, -65.9177)
  arc A1001 (-50.6991, -85.4677) -> (-51.1991, -84.9677) centre (-51.1991, -85.4677) ccw
  arc A1002 (27.3822, -41.8177) -> (27.8822, -41.3177) centre (27.3822, -41.3177) ccw
  arc A1003 (113.6072, -9.2677) -> (113.1072, -8.7677) centre (113.1072, -9.2677) ccw
  arc A1004 (-48.0303, -79.4177) -> (-47.5303, -79.9177) centre (-47.5303, -79.4177) ccw
  line L1041 (46.9322, -28.3177) -> (46.9322, -41.3177)
  arc A1005 (-20.2428, -3.7177) -> (-19.7428, -3.2177) centre (-20.2428, -3.2177) ccw
  line L1042 (4.0697, -66.4177) -> (4.0697, -79.4177)
  arc A1006 (75.7947, -60.3677) -> (76.2947, -60.8677) centre (76.2947, -60.3677) ccw
  arc A1007 (4.0697, -66.4177) -> (3.5697, -65.9177) centre (3.5697, -66.4177) ccw
  arc A1008 (194.8572, -98.4677) -> (195.3572, -98.9677) centre (195.3572, -98.4677) ccw
  line L1043 (80.5572, 9.7823) -> (80.5572, -3.2177)
  line L1044 (4.3572, 9.7823) -> (4.3572, -3.2177)
  line L1045 (27.8822, -28.3177) -> (27.8822, -41.3177)
  line L1046 (-63.0486, -66.9177) -> (-57.0486, -66.9177)
  arc A1009 (61.5072, -3.2177) -> (62.0072, -3.7177) centre (62.0072, -3.2177) ccw
  arc A1010 (-51.1991, -98.9677) -> (-50.6991, -98.4677) centre (-51.1991, -98.4677) ccw
  line L1047 (-8.9491, -86.4677) -> (-8.9491, -100.4677)
  line L1048 (175.8072, -66.4177) -> (175.8072, -79.4177)
  arc A1011 (84.5509, -85.9677) -> (84.0509, -86.4677) centre (84.5509, -86.4677) ccw
  arc A1012 (94.5572, -9.2677) -> (94.0572, -8.7677) centre (94.0572, -9.2677) ccw
  line L1049 (166.7822, -22.7677) -> (179.7822, -22.7677)
  line L1050 (176.3072, -98.9677) -> (189.3072, -98.9677)
  line L1051 (66.7697, -79.9177) -> (79.7697, -79.9177)
  line L1052 (195.3572, -60.8677) -> (208.3572, -60.8677)
  arc A1013 (-14.1928, 10.2823) -> (-14.6928, 9.7823) centre (-14.1928, 9.7823) ccw
  arc A1014 (100.1072, 10.2823) -> (99.6072, 9.7823) centre (100.1072, 9.7823) ccw
  arc A1015 (81.0572, 10.2823) -> (80.5572, 9.7823) centre (81.0572, 9.7823) ccw
  line L1053 (-0.6928, 9.7823) -> (-0.6928, -3.2177)
  line L1054 (137.7072, -9.2677) -> (137.7072, -22.2677)
  line L1055 (157.2572, -98.9677) -> (170.2572, -98.9677)
  line L1056 (179.8389, -62.8677) -> (185.8389, -62.8677)
  arc A1016 (62.0072, 10.2823) -> (61.5072, 9.7823) centre (62.0072, 9.7823) ccw
  arc A1017 (-78.4866, -65.9177) -> (-78.9866, -66.4177) centre (-78.4866, -66.4177) ccw
  line L1057 (33.4322, -27.8177) -> (46.4322, -27.8177)
  arc A1018 (-19.4553, -60.3677) -> (-18.9553, -60.8677) centre (-18.9553, -60.3677) ccw
  arc A1019 (9.6197, -65.9177) -> (9.1197, -66.4177) centre (9.6197, -66.4177) ccw
  line L1058 (84.5509, -100.9677) -> (90.5509, -100.9677)
  line L1059 (-83.2491, -60.8677) -> (-70.2491, -60.8677)
  arc A1020 (119.1572, 10.2823) -> (118.6572, 9.7823) centre (119.1572, 9.7823) ccw
  arc A1021 (-47.5303, -65.9177) -> (-48.0303, -66.4177) centre (-47.5303, -66.4177) ccw
  arc A1022 (23.4072, -22.2677) -> (23.9072, -22.7677) centre (23.9072, -22.2677) ccw
  arc A1023 (127.3947, -60.8677) -> (127.8947, -60.3677) centre (127.3947, -60.3677) ccw
  line L1060 (118.6572, -9.2677) -> (118.6572, -22.2677)
  line L1061 (62.0072, 10.2823) -> (75.0072, 10.2823)
  line L1062 (175.8072, -85.4677) -> (175.8072, -98.4677)
  line L1063 (-14.6928, 9.7823) -> (-14.6928, -3.2177)
  arc A1024 (113.8947, -60.3677) -> (114.3947, -60.8677) centre (114.3947, -60.3677) ccw
  arc A1025 (32.6447, -47.3677) -> (32.1447, -46.8677) centre (32.1447, -47.3677) ccw
  arc A1026 (185.8389, -62.8677) -> (186.3389, -62.3677) centre (185.8389, -62.3677) ccw
  line L1064 (90.0822, -28.3177) -> (90.0822, -41.3177)
  line L1065 (99.6072, -85.4677) -> (99.6072, -98.4677)
  line L1066 (195.3572, -98.9677) -> (208.3572, -98.9677)
  line L1067 (-52.2928, -8.7677) -> (-39.2928, -8.7677)
  arc A1027 (80.5572, -22.2677) -> (81.0572, -22.7677) centre (81.0572, -22.2677) ccw
  line L1068 (-14.1928, 10.2823) -> (-1.1928, 10.2823)
  arc A1028 (113.6072, 9.7823) -> (113.1072, 10.2823) centre (113.1072, 9.7823) ccw
  arc A1029 (38.1947, -46.8677) -> (37.6947, -47.3677) centre (38.1947, -47.3677) ccw
  arc A1030 (-40.3866, -84.9677) -> (-40.8866, -85.4677) centre (-40.3866, -85.4677) ccw
  line L1069 (85.3197, -66.4177) -> (85.3197, -79.4177)
  arc A1031 (132.1572, -98.9677) -> (132.6572, -98.4677) centre (132.1572, -98.4677) ccw
  arc A1032 (46.4322, -41.8177) -> (46.9322, -41.3177) centre (46.4322, -41.3177) ccw
  line L1070 (150.1134, -65.9177) -> (163.1134, -65.9177)
  line L1071 (176.3072, -79.9177) -> (189.3072, -79.9177)
  line L1072 (113.6072, -9.2677) -> (113.6072, -22.2677)
  arc A1033 (-57.5553, -60.3677) -> (-57.0553, -60.8677) centre (-57.0553, -60.3677) ccw
  arc A1034 (75.0072, -22.7677) -> (75.5072, -22.2677) centre (75.0072, -22.2677) ccw
  arc A1035 (52.4822, -27.8177) -> (51.9822, -28.3177) centre (52.4822, -28.3177) ccw
  arc A1036 (179.3389, -62.3677) -> (179.8389, -62.8677) centre (179.8389, -62.3677) ccw
  arc A1037 (113.1072, -3.7177) -> (113.6072, -3.2177) centre (113.1072, -3.2177) ccw
  arc A1038 (-38.5053, -60.3677) -> (-38.0053, -60.8677) centre (-38.0053, -60.3677) ccw
  arc A1039 (157.2572, -84.9677) -> (156.7572, -85.4677) centre (157.2572, -85.4677) ccw
  arc A1040 (94.5572, 9.7823) -> (94.0572, 10.2823) centre (94.0572, 9.7823) ccw
  arc A1041 (46.9322, -28.3177) -> (46.4322, -27.8177) centre (46.4322, -28.3177) ccw
  arc A1042 (-52.2928, 10.2823) -> (-52.7928, 9.7823) centre (-52.2928, 9.7823) ccw
  arc A1043 (-70.2491, -60.8677) -> (-69.7491, -60.3677) centre (-70.2491, -60.3677) ccw
  arc A1044 (-14.1928, -8.7677) -> (-14.6928, -9.2677) centre (-14.1928, -9.2677) ccw